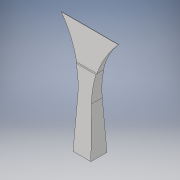
# Autodesk Inventor part: bachi
Saved by Autodesk Inventor 2019 (Build 230136000, 136)
## iProperties
Created: 2020-07-09
Part Number: bachi
Material: Типовые
Document SubType Name: Modeling
Designer: stepa
Density: 1 g/cm^3
Appearance: По умолчанию
Author: stepa
Autodesk Inventor part; units mm, degrees
ref_plane "YZ Plane" through (0, 0, 0) normal (1, 0, 0) x (0, 1, 0)
ref_plane "XZ Plane" through (0, 0, 0) normal (0, 1, 0) x (-1, 0, 0)
ref_plane "XY Plane" through (0, 0, 0) normal (0, 0, 1) x (1, 0, 0)
sketch "Эскиз1" plane through (0, 0, 0) normal (0, 0, 1) x (1, 0, 0)
  line L0 (-15, 0) -> (15, 0)
  line L1 (0, 120) -> (0, 125)
  line L2 (0, 125) -> (0, 180)
  line L3 (-48, 180) -> (48, 180)
  line L4 (-17, 125) -> (17, 125)
  line L5 (-15, 120) -> (15, 120)
  line L6 (0, 0) -> (0, 80)
  line L7 (0, 80) -> (0, 120)
  line L8 (-11.5, 80) -> (11.5, 80)
  line L9 (15, 0) -> (11.5, 80)
  line L10 (-15, 0) -> (-11.5, 80)
  arc A0 (17, 125) -> (11.5, 80) centre (149.09, 86.0196) ccw
  arc A1 (48, 180) -> (17, 125) centre (151.9429, 85.1776) ccw
  arc A2 (-11.5, 80) -> (-17, 125) centre (-149.09, 86.0196) ccw
  arc A3 (-17, 125) -> (-48, 180) centre (-151.9429, 85.1776) ccw
  dimension "d0" = 30
  dimension "d2" = 5
  dimension "d3" = 55
  dimension "d4" = 96
  dimension "d5" = 34
  dimension "d6" = 30
  dimension "d7" = 80
  dimension "d8" = 40
  dimension "d9" = 23
  constraints: 22 end point, 8 point on circle, 5 horizontal, 5 midpoint, 4 centre point, 4 tangent, 2 vertical, 1 collinear, 1 point on line
  measures "d0" distance of L0.start L0.end
  measures "d2" distance of L1.end L1.start
  measures "d3" distance of L2.end L1.end
  measures "d4" distance of L3.start L3.end
  measures "d5" distance of L4.start L4.end
  measures "d6" distance of L5.start L5.end
  measures "d7" distance of L6.end L6.start
  measures "d8" distance of L6.end L1.start
  measures "d9" distance of L8.start L8.end
extrude "Выдавливание1" add sketch "Эскиз1" along normal blind 27
sketch "Эскиз2" plane through (0, 0, 0) normal (1, 0, 0) x (0, 1, 0)
  line L0 (80, 0) -> (0, 0) projected
  line L1 (0, 0) -> (0, 27) projected
  line L2 (80, 27) -> (0, 27) projected
  line L3 (80, 0) -> (80, 27) projected
  line L4 (125, 0) -> (80, 0) projected
  line L5 (80, 0) -> (80, 27) projected
  line L6 (125, 27) -> (80, 27) projected
  line L7 (125, 0) -> (125, 27) projected
  line L8 (180, 0) -> (125, 0) projected
  line L9 (125, 0) -> (125, 27) projected
  line L10 (180, 27) -> (125, 27) projected
  line L11 (180, 0) -> (180, 27) projected
  line L12 (125, 7) -> (125, 20)
  line L13 (125, 0) -> (125, 27) projected
  line L14 (125, 7) -> (0, 0)
  line L15 (0, 27) -> (125, 20)
  line L16 (125, 8) -> (125, 19)
  line L17 (180, 13.25) -> (180, 13.75)
  line L18 (180, 0) -> (180, 27) projected
  line L19 (125, 8) -> (180, 13.25)
  line L20 (180, 13.75) -> (125, 19)
  point P0 (125, 13.5)
  point P1 (125, 13.5)
  point P2 (180, 13.5)
  dimension "d12" = 13
  dimension "d13" = 11
  dimension "d14" = 0.5
  constraints: 14 end point, 6 midpoint, 2 point on line, 2 vertical
  measures "d12" distance of L12.start L12.end
  measures "d13" distance of L16.start L16.end
  measures "d14" distance of L17.start L17.end
extrude "Выдавливание2" cut sketch "Эскиз2" along normal mid plane 100 contours L1 L15 L3 L14 | L3 L15 L7 L14 | L7 L20 L11 L19 keep common part
chamfer "Фаска1" distance 1 angle 45 2 edges at (0, 125, 7) (0, 125, 20)
equation "\"d6\" = d0"
